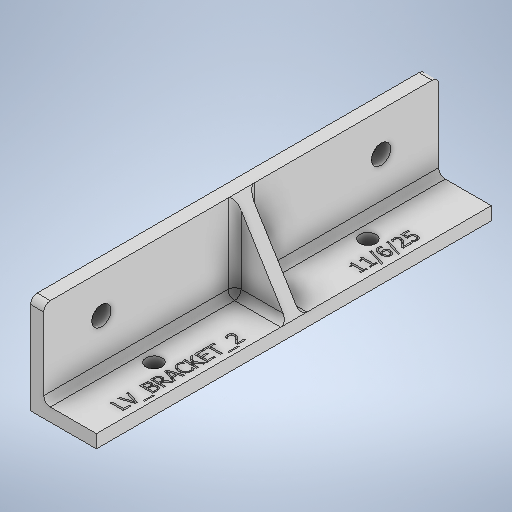
# Autodesk Inventor part: LV_Bracket_2
Saved by Autodesk Inventor 2025 (Build 290162000, 162)
## iProperties
Created: 2025-05-19
Part Number: LV_Bracket_2
Material: Generic
Document SubType Name: Modeling
Designer: mumin
Density: 1 g/cm^3
Appearance: Default
Author: mumin
Autodesk Inventor part; units mm, degrees
ref_plane "YZ Plane" through (0, 0, 0) normal (1, 0, 0) x (0, 1, 0)
ref_plane "XZ Plane" through (0, 0, 0) normal (0, 1, 0) x (-1, 0, 0)
ref_plane "XY Plane" through (0, 0, 0) normal (0, 0, 1) x (1, 0, 0)
sketch "Sketch1" plane through (0, 0, 0) normal (0, 0, 1) x (1, 0, 0)
  line L0 (-4, 26) -> (-4, -4)
  line L1 (-4, -4) -> (16, -4)
  line L2 (16, -4) -> (16, 0)
  line L3 (16, 0) -> (0, 0)
  line L4 (0, 0) -> (0, 26)
  line L5 (0, 26) -> (-4, 26)
  point P0 (0, 0)
  dimension "d0" = 30
  dimension "d1" = 20
  dimension "d2" = 4
  dimension "d3" = 4
  constraints: 12 end point, 5 perpendicular, 1 vertical
  measures "d0" distance of L0.start L0.end
  measures "d1" distance of L0.end L1.end
  measures "d2" distance of L1.end L2.end
  measures "d3" distance between parallel lines of L4 L0
extrude "Base" add sketch "Sketch1" along normal mid plane 120
sketch "Sketch2" plane through (0, 0, 0) normal (0, 0, 1) x (1, 0, 0)
  line L0 (0, 0) -> (0, 26) projected
  line L1 (16, -4) -> (16, 0) projected
  line L2 (0, 26) -> (16, 0)
  line L3 (16, 0) -> (0, 0)
  constraints: 4 end point, 1 perpendicular
extrude "Center Truss" add sketch "Sketch2" along normal mid plane 4
fillet "Fillet1" radius 2 8 edges at (0, 0, 31) (0, 0, -31) (0, 13, 2) (8, 0, 2) (0, 13, -2) (8, 0, -2) (-2, 26, 60) (-2, 26, -60)
sketch "Sketch3" plane through (0, 2, 4) normal (1, 0, 0) x (0, 0, -1)
  line L0 (64, -6) -> (-56, -6) projected
  line L1 (8, 24) -> (0, 24) projected
  point P0 (4, -2)
  point P1 (-38.5, 12.28)
  point P2 (4, 24)
  dimension "d19" = 18.28
  dimension "d20" = 42.5
  constraints: 1 midpoint
  measures "d19" distance from line of L0 point (-38.5, 12.28)
  measures "d20" horizontal distance of point (4, 24) point (-38.5, 12.28)
hole "LV Mount Hole" at (0, 14.28, 42.5) direction (-1, 0, 0) diameter 5.9 depth 4 tip angle 118
mirror "Mirror1" about plane through (0, 0, 0) normal (0, 0, 1) of "LV Mount Hole"
sketch "Sketch4" plane through (2, 0, 4) normal (0, 1, 0) x (1, 0, 0)
  line L0 (14, 0) -> (14, -56) projected
  line L1 (14, 8) -> (14, 0) projected
  point P0 (-2, 4)
  point P1 (4, -28.5)
  point P2 (14, -50)
  point P3 (14, 4)
  dimension "d28" = 10
  dimension "d29" = 32.5
  constraints: 1 midpoint
  measures "d28" distance from line of L0 point (4, -28.5)
  measures "d29" vertical distance of point (14, 4) point (4, -28.5)
hole "80/20 Mount Hole" at (6, 0, 32.5) direction (0, -1, 0) diameter 4.9 depth 4 tip angle 118
mirror "Mirror2" about plane through (0, 0, 0) normal (0, 0, 1) of "80/20 Mount Hole"
sketch "Sketch5" plane through (-4, -4, -60) normal (-1, 0, 0) x (0, 0, 1)
  circle A0 centre (89, 18.28) radius 1.85
  line L0 (120, 28) -> (120, 0) projected
  circle A1 centre (29.5, 18.28) radius 1.85
  circle A2 centre (17.5, 18.28) radius 2.95 projected
  point P0 (60, 4)
  dimension "d31" = 3.7
  dimension "d32" = 31
  dimension "d33" = 3.7
  dimension "d34" = 12
  constraints: 2 centre point
  measures "d31" diameter of A0
  measures "d32" distance from line of L0 A0.centre
  measures "d33" diameter of A1
  measures "d34" distance of A1.centre A2.centre
extrude "Alignment Pins" add sketch "Sketch5" along normal blind 3 contours A0 | A1
fillet "Fillet2" radius 1 2 edges at (-7, 14.28, -32.35) (-7, 14.28, 27.15)
sketch "Sketch6" plane through (2, 0, 60) normal (0, 1, 0) x (1, 0, 0)
  line L0 (7.8938, 9.7827) -> (7.8938, 38.5979) construction
  line L1 (7.8938, 38.5979) -> (11.6186, 38.5979) construction
  line L2 (11.6186, 38.5979) -> (11.6186, 9.7827) construction
  line L3 (11.6186, 9.7827) -> (7.8938, 9.7827) construction
  line L4 (7.6408, 81.9717) -> (7.6408, 104.1889) construction
  line L5 (7.6408, 104.1889) -> (12.6878, 104.1889) construction
  line L6 (12.6878, 104.1889) -> (12.6878, 81.9717) construction
  line L7 (12.6878, 81.9717) -> (7.6408, 81.9717) construction
  line L8 (11.9781, 12.5056) -> (11.9781, 10.1879)
  line L9 (11.9781, 10.1879) -> (7.9781, 10.1879)
  line L10 (7.9781, 10.1879) -> (7.9781, 10.7195)
  line L11 (7.9781, 10.7195) -> (11.5049, 10.7195)
  line L12 (11.5049, 10.7195) -> (11.5049, 12.5056)
  line L13 (11.5049, 12.5056) -> (11.9781, 12.5056)
  line L14 (7.9781, 15.8248) -> (11.9781, 14.4472)
  line L15 (11.9781, 14.4472) -> (11.9781, 13.8735)
  line L16 (11.9781, 13.8735) -> (7.9781, 12.4958)
  line L17 (7.9781, 12.4958) -> (7.9781, 13.0663)
  line L18 (7.9781, 13.0663) -> (11.3006, 14.1749)
  line L19 (11.3006, 14.1749) -> (7.9781, 15.2835)
  line L20 (7.9781, 15.2835) -> (7.9781, 15.8248)
  line L21 (12.782, 18.8459) -> (12.782, 15.76)
  line L22 (12.782, 15.76) -> (12.4352, 15.76)
  line L23 (12.4352, 15.76) -> (12.4352, 18.8459)
  line L24 (12.4352, 18.8459) -> (12.782, 18.8459)
  spline S0 degree 2 poles (10.7496, 21.9221) (11.0478, 21.9221) (11.5049, 21.6952) (11.654, 21.5072) knots 0 0 0 1 2 2 2
  spline S1 degree 2 poles (11.654, 21.5072) (11.829, 21.2803) (11.9781, 20.7649) (11.9781, 20.3564) knots 0 0 0 1 2 2 2
  line L25 (11.9781, 20.3564) -> (11.9781, 19.209)
  line L26 (11.9781, 19.209) -> (7.9781, 19.209)
  line L27 (7.9781, 19.209) -> (7.9781, 20.2689)
  spline S2 degree 2 poles (7.9781, 20.2689) (7.9781, 20.6968) (8.0332, 21.1247) (8.1402, 21.3192) knots 0 0 0 1 2 2 2
  spline S3 degree 2 poles (8.1402, 21.3192) (8.2536, 21.5363) (8.6264, 21.7341) (8.8793, 21.7341) knots 0 0 0 1 2 2 2
  spline S4 degree 2 poles (8.8793, 21.7341) (9.1613, 21.7341) (9.6086, 21.4359) (9.735, 21.1733) knots 0 0 0 1 2 2 2
  line L28 (9.735, 21.1733) -> (9.7545, 21.1733)
  spline S5 degree 2 poles (9.7545, 21.1733) (9.8517, 21.5299) (10.3671, 21.9221) (10.7496, 21.9221) knots 0 0 0 1 2 2 2
  spline S6 degree 2 poles (10.7723, 21.3678) (10.5454, 21.3678) (10.2536, 21.2381) (10.1499, 21.0436) knots 0 0 0 1 2 2 2
  spline S7 degree 2 poles (10.1499, 21.0436) (10.0851, 20.9172) (10.0462, 20.619) (10.0462, 20.3435) knots 0 0 0 1 2 2 2
  line L29 (10.0462, 20.3435) -> (10.0462, 19.7406)
  line L30 (10.0462, 19.7406) -> (11.5243, 19.7406)
  line L31 (11.5243, 19.7406) -> (11.5243, 20.1717)
  spline S8 degree 2 poles (11.5243, 20.1717) (11.5243, 20.5218) (11.4595, 20.9237) (11.3558, 21.0793) knots 0 0 0 1 2 2 2
  spline S9 degree 2 poles (11.3558, 21.0793) (11.2488, 21.2284) (10.983, 21.3678) (10.7723, 21.3678) knots 0 0 0 1 2 2 2
  spline S10 degree 2 poles (8.9538, 21.1798) (8.8112, 21.1798) (8.5972, 21.0825) (8.5357, 20.9756) knots 0 0 0 1 2 2 2
  spline S11 degree 2 poles (8.5357, 20.9756) (8.4643, 20.8459) (8.4319, 20.5315) (8.4319, 20.2495) knots 0 0 0 1 2 2 2
  line L32 (8.4319, 20.2495) -> (8.4319, 19.7406)
  line L33 (8.4319, 19.7406) -> (9.6021, 19.7406)
  line L34 (9.6021, 19.7406) -> (9.6021, 20.3435)
  spline S12 degree 2 poles (9.6021, 20.3435) (9.6021, 20.5931) (9.5502, 20.8297) (9.4692, 20.9561) knots 0 0 0 1 2 2 2
  spline S13 degree 2 poles (9.4692, 20.9561) (9.3914, 21.0793) (9.1418, 21.1798) (8.9538, 21.1798) knots 0 0 0 1 2 2 2
  line L35 (11.9781, 25.5461) -> (11.9781, 24.8556)
  line L36 (11.9781, 24.8556) -> (10.3865, 23.5914)
  line L37 (10.3865, 23.5914) -> (10.3865, 22.982)
  line L38 (10.3865, 22.982) -> (11.9781, 22.982)
  line L39 (11.9781, 22.982) -> (11.9781, 22.4504)
  line L40 (11.9781, 22.4504) -> (7.9781, 22.4504)
  line L41 (7.9781, 22.4504) -> (7.9781, 23.4812)
  spline S14 degree 2 poles (7.9781, 23.4812) (7.9781, 23.8248) (8.0527, 24.2884) (8.1888, 24.4991) knots 0 0 0 1 2 2 2
  spline S15 degree 2 poles (8.1888, 24.4991) (8.325, 24.7098) (8.7496, 24.9529) (9.064, 24.9529) knots 0 0 0 1 2 2 2
  spline S16 degree 2 poles (9.064, 24.9529) (9.5016, 24.9529) (10.0948, 24.5056) (10.2374, 24.1231) knots 0 0 0 1 2 2 2
  line L42 (10.2374, 24.1231) -> (11.9781, 25.5461)
  spline S17 degree 2 poles (9.1062, 24.3986) (8.9311, 24.3986) (8.6621, 24.2754) (8.5746, 24.1457) knots 0 0 0 1 2 2 2
  spline S18 degree 2 poles (8.5746, 24.1457) (8.5, 24.0323) (8.4384, 23.7308) (8.4384, 23.5104) knots 0 0 0 1 2 2 2
  line L43 (8.4384, 23.5104) -> (8.4384, 22.982)
  line L44 (8.4384, 22.982) -> (9.9425, 22.982)
  line L45 (9.9425, 22.982) -> (9.9425, 23.4488)
  spline S19 degree 2 poles (9.9425, 23.4488) (9.9425, 23.679) (9.8614, 24.0453) (9.735, 24.1717) knots 0 0 0 1 2 2 2
  spline S20 degree 2 poles (9.735, 24.1717) (9.6248, 24.2884) (9.3136, 24.3986) (9.1062, 24.3986) knots 0 0 0 1 2 2 2
  line L46 (11.9781, 25.4326) -> (7.9781, 26.7811)
  line L47 (7.9781, 26.7811) -> (7.9781, 27.4359)
  line L48 (7.9781, 27.4359) -> (11.9781, 28.7843)
  line L49 (11.9781, 28.7843) -> (11.9781, 28.2235)
  line L50 (11.9781, 28.2235) -> (10.8598, 27.8605)
  line L51 (10.8598, 27.8605) -> (10.8598, 26.3338)
  line L52 (10.8598, 26.3338) -> (11.9781, 25.9707)
  line L53 (11.9781, 25.9707) -> (11.9781, 25.4326)
  line L54 (10.406, 27.7146) -> (8.5227, 27.0955)
  line L55 (8.5227, 27.0955) -> (10.406, 26.4796)
  line L56 (10.406, 26.4796) -> (10.406, 27.7146)
  spline S21 degree 2 poles (12.0494, 30.726) (12.0494, 30.337) (11.7869, 29.679) (11.5243, 29.4391) knots 0 0 0 1 2 2 2
  spline S22 degree 2 poles (11.5243, 29.4391) (11.265, 29.1992) (10.487, 28.9367) (9.9814, 28.9367) knots 0 0 0 1 2 2 2
  spline S23 degree 2 poles (9.9814, 28.9367) (9.4789, 28.9367) (8.7334, 29.1927) (8.4579, 29.4359) knots 0 0 0 1 2 2 2
  spline S24 degree 2 poles (8.4579, 29.4359) (8.1888, 29.6757) (7.9068, 30.3305) (7.9068, 30.7357) knots 0 0 0 1 2 2 2
  spline S25 degree 2 poles (7.9068, 30.7357) (7.9068, 30.9367) (7.9652, 31.29) (8.0105, 31.4391) knots 0 0 0 1 2 2 2
  spline S26 degree 2 poles (8.0105, 31.4391) (8.0527, 31.5688) (8.1726, 31.8378) (8.2439, 31.9707) knots 0 0 0 1 2 2 2
  line L57 (8.2439, 31.9707) -> (8.8857, 31.9707)
  line L58 (8.8857, 31.9707) -> (8.8857, 31.9286)
  spline S27 degree 2 poles (8.8857, 31.9286) (8.8209, 31.8573) (8.6394, 31.6368) (8.5519, 31.478) knots 0 0 0 1 2 2 2
  spline S28 degree 2 poles (8.5519, 31.478) (8.4676, 31.3256) (8.3606, 30.9658) (8.3606, 30.7325) knots 0 0 0 1 2 2 2
  spline S29 degree 2 poles (8.3606, 30.7325) (8.3606, 30.4764) (8.5713, 30.0193) (8.7723, 29.8475) knots 0 0 0 1 2 2 2
  spline S30 degree 2 poles (8.7723, 29.8475) (8.9765, 29.679) (9.5956, 29.491) (9.9814, 29.491) knots 0 0 0 1 2 2 2
  spline S31 degree 2 poles (9.9814, 29.491) (10.393, 29.491) (10.9862, 29.6887) (11.1904, 29.8605) knots 0 0 0 1 2 2 2
  spline S32 degree 2 poles (11.1904, 29.8605) (11.3882, 30.0291) (11.5891, 30.4796) (11.5891, 30.7325) knots 0 0 0 1 2 2 2
  spline S33 degree 2 poles (11.5891, 30.7325) (11.5891, 30.9626) (11.4757, 31.3548) (11.3914, 31.5072) knots 0 0 0 1 2 2 2
  spline S34 degree 2 poles (11.3914, 31.5072) (11.3071, 31.653) (11.1321, 31.8702) (11.0705, 31.9318) knots 0 0 0 1 2 2 2
  line L59 (11.0705, 31.9318) -> (11.0705, 31.9707)
  line L60 (11.0705, 31.9707) -> (11.7058, 31.9707)
  spline S35 degree 2 poles (11.7058, 31.9707) (11.7674, 31.8378) (11.8809, 31.6044) (11.9327, 31.4391) knots 0 0 0 1 2 2 2
  spline S36 degree 2 poles (11.9327, 31.4391) (11.9911, 31.2641) (12.0494, 30.9658) (12.0494, 30.726) knots 0 0 0 1 2 2 2
  line L61 (11.9781, 35.384) -> (11.9781, 34.6936)
  line L62 (11.9781, 34.6936) -> (10.1175, 33.2316)
  line L63 (10.1175, 33.2316) -> (10.3801, 32.9983)
  line L64 (10.3801, 32.9983) -> (11.9781, 32.9983)
  line L65 (11.9781, 32.9983) -> (11.9781, 32.4667)
  line L66 (11.9781, 32.4667) -> (7.9781, 32.4667)
  line L67 (7.9781, 32.4667) -> (7.9781, 32.9983)
  line L68 (7.9781, 32.9983) -> (9.816, 32.9983)
  line L69 (9.816, 32.9983) -> (7.9781, 34.6385)
  line L70 (7.9781, 34.6385) -> (7.9781, 35.2867)
  line L71 (7.9781, 35.2867) -> (9.7642, 33.6303)
  line L72 (9.7642, 33.6303) -> (11.9781, 35.384)
  line L73 (11.9781, 35.7017) -> (7.9781, 35.7017)
  line L74 (7.9781, 35.7017) -> (7.9781, 38.2041)
  line L75 (7.9781, 38.2041) -> (8.4514, 38.2041)
  line L76 (8.4514, 38.2041) -> (8.4514, 36.2333)
  line L77 (8.4514, 36.2333) -> (9.547, 36.2333)
  line L78 (9.547, 36.2333) -> (9.547, 38.0712)
  line L79 (9.547, 38.0712) -> (10.0203, 38.0712)
  line L80 (10.0203, 38.0712) -> (10.0203, 36.2333)
  line L81 (10.0203, 36.2333) -> (11.5049, 36.2333)
  line L82 (11.5049, 36.2333) -> (11.5049, 38.2041)
  line L83 (11.5049, 38.2041) -> (11.9781, 38.2041)
  line L84 (11.9781, 38.2041) -> (11.9781, 35.7017)
  line L85 (11.9781, 39.7211) -> (8.4514, 39.7211)
  line L86 (8.4514, 39.7211) -> (8.4514, 38.3791)
  line L87 (8.4514, 38.3791) -> (7.9781, 38.3791)
  line L88 (7.9781, 38.3791) -> (7.9781, 41.5947)
  line L89 (7.9781, 41.5947) -> (8.4514, 41.5947)
  line L90 (8.4514, 41.5947) -> (8.4514, 40.2527)
  line L91 (8.4514, 40.2527) -> (11.9781, 40.2527)
  line L92 (11.9781, 40.2527) -> (11.9781, 39.7211)
  line L93 (12.782, 44.6385) -> (12.782, 41.5526)
  line L94 (12.782, 41.5526) -> (12.4352, 41.5526)
  line L95 (12.4352, 41.5526) -> (12.4352, 44.6385)
  line L96 (12.4352, 44.6385) -> (12.782, 44.6385)
  line L97 (11.9781, 47.3548) -> (11.9781, 44.888)
  line L98 (11.9781, 44.888) -> (11.4109, 44.888)
  spline S37 degree 2 poles (11.4109, 44.888) (11.1613, 45.1538) (10.6977, 45.6271) (10.4481, 45.854) knots 0 0 0 1 2 2 2
  spline S38 degree 2 poles (10.4481, 45.854) (9.9457, 46.3111) (9.3428, 46.6449) (9.0219, 46.6449) knots 0 0 0 1 2 2 2
  spline S39 degree 2 poles (9.0219, 46.6449) (8.8533, 46.6449) (8.6005, 46.5412) (8.5194, 46.4472) knots 0 0 0 1 2 2 2
  spline S40 degree 2 poles (8.5194, 46.4472) (8.4384, 46.3532) (8.3574, 46.1068) (8.3574, 45.9577) knots 0 0 0 1 2 2 2
  spline S41 degree 2 poles (8.3574, 45.9577) (8.3574, 45.8151) (8.4287, 45.5234) (8.4838, 45.3905) knots 0 0 0 1 2 2 2
  spline S42 degree 2 poles (8.4838, 45.3905) (8.5292, 45.277) (8.6588, 45.0663) (8.7042, 45.0015) knots 0 0 0 1 2 2 2
  line L99 (8.7042, 45.0015) -> (8.7042, 44.9723)
  line L100 (8.7042, 44.9723) -> (8.1337, 44.9723)
  spline S43 degree 2 poles (8.1337, 44.9723) (8.0527, 45.1376) (7.8938, 45.7308) (7.8938, 45.9966) knots 0 0 0 1 2 2 2
  spline S44 degree 2 poles (7.8938, 45.9966) (7.8938, 46.5574) (8.487, 47.1895) (8.9927, 47.1895) knots 0 0 0 1 2 2 2
  spline S45 degree 2 poles (8.9927, 47.1895) (9.2293, 47.1895) (9.6248, 47.0793) (9.7934, 46.9821) knots 0 0 0 1 2 2 2
  spline S46 degree 2 poles (9.7934, 46.9821) (9.9684, 46.8848) (10.312, 46.6028) (10.4773, 46.4472) knots 0 0 0 1 2 2 2
  spline S47 degree 2 poles (10.4773, 46.4472) (10.7528, 46.1944) (11.3428, 45.5752) (11.5146, 45.3905) knots 0 0 0 1 2 2 2
  line L101 (11.5146, 45.3905) -> (11.5146, 47.3548)
  line L102 (11.5146, 47.3548) -> (11.9781, 47.3548)
  line L103 (11.8191, 84.5292) -> (11.8191, 82.5778)
  line L104 (11.8191, 82.5778) -> (11.4106, 82.5778)
  line L105 (11.4106, 82.5778) -> (11.4106, 83.3039)
  line L106 (11.4106, 83.3039) -> (8.7299, 83.3039)
  line L107 (8.7299, 83.3039) -> (8.7299, 82.5778)
  line L108 (8.7299, 82.5778) -> (8.3636, 82.5778)
  spline S48 degree 2 poles (8.3636, 82.5778) (8.3636, 82.9895) (8.1302, 83.3785) (7.8061, 83.4044) knots 0 0 0 1 2 2 2
  line L109 (7.8061, 83.4044) -> (7.8061, 83.8193)
  line L110 (7.8061, 83.8193) -> (11.4106, 83.8193)
  line L111 (11.4106, 83.8193) -> (11.4106, 84.5292)
  line L112 (11.4106, 84.5292) -> (11.8191, 84.5292)
  line L113 (11.8191, 87.5308) -> (11.8191, 85.5795)
  line L114 (11.8191, 85.5795) -> (11.4106, 85.5795)
  line L115 (11.4106, 85.5795) -> (11.4106, 86.3056)
  line L116 (11.4106, 86.3056) -> (8.7299, 86.3056)
  line L117 (8.7299, 86.3056) -> (8.7299, 85.5795)
  line L118 (8.7299, 85.5795) -> (8.3636, 85.5795)
  spline S49 degree 2 poles (8.3636, 85.5795) (8.3636, 85.9911) (8.1302, 86.3801) (7.8061, 86.406) knots 0 0 0 1 2 2 2
  line L119 (7.8061, 86.406) -> (7.8061, 86.821)
  line L120 (7.8061, 86.821) -> (11.4106, 86.821)
  line L121 (11.4106, 86.821) -> (11.4106, 87.5308)
  line L122 (11.4106, 87.5308) -> (11.8191, 87.5308)
  line L123 (7.6408, 89.9295) -> (12.6878, 88.3639)
  line L124 (12.6878, 88.3639) -> (12.6878, 87.9101)
  line L125 (12.6878, 87.9101) -> (7.6408, 89.4693)
  line L126 (7.6408, 89.4693) -> (7.6408, 89.9295)
  spline S50 degree 2 poles (10.5225, 92.8988) (10.8304, 92.8988) (11.3523, 92.6945) (11.5273, 92.5227) knots 0 0 0 1 2 2 2
  spline S51 degree 2 poles (11.5273, 92.5227) (11.7121, 92.3445) (11.9033, 91.8971) (11.9033, 91.6281) knots 0 0 0 1 2 2 2
  spline S52 degree 2 poles (11.9033, 91.6281) (11.9033, 91.359) (11.7218, 90.915) (11.5403, 90.7464) knots 0 0 0 1 2 2 2
  spline S53 degree 2 poles (11.5403, 90.7464) (11.3231, 90.5389) (10.5938, 90.3056) (10.0622, 90.3056) knots 0 0 0 1 2 2 2
  spline S54 degree 2 poles (10.0622, 90.3056) (9.5403, 90.3056) (8.7007, 90.5195) (8.3896, 90.7432) knots 0 0 0 1 2 2 2
  spline S55 degree 2 poles (8.3896, 90.7432) (8.0849, 90.9603) (7.7445, 91.6475) (7.7445, 92.0981) knots 0 0 0 1 2 2 2
  spline S56 degree 2 poles (7.7445, 92.0981) (7.7445, 92.231) (7.7704, 92.4644) (7.7996, 92.5519) knots 0 0 0 1 2 2 2
  line L127 (7.7996, 92.5519) -> (8.315, 92.5519)
  line L128 (8.315, 92.5519) -> (8.315, 92.5292)
  spline S57 degree 2 poles (8.315, 92.5292) (8.2761, 92.4547) (8.208, 92.1824) (8.208, 92.0268) knots 0 0 0 1 2 2 2
  spline S58 degree 2 poles (8.208, 92.0268) (8.208, 91.5276) (8.8823, 90.915) (9.5435, 90.8566) knots 0 0 0 1 2 2 2
  spline S59 degree 2 poles (9.5435, 90.8566) (9.4106, 91.0479) (9.2648, 91.4498) (9.2648, 91.6897) knots 0 0 0 1 2 2 2
  spline S60 degree 2 poles (9.2648, 91.6897) (9.2648, 91.9231) (9.3588, 92.2731) (9.5014, 92.4644) knots 0 0 0 1 2 2 2
  spline S61 degree 2 poles (9.5014, 92.4644) (9.6667, 92.6848) (10.1789, 92.8988) (10.5225, 92.8988) knots 0 0 0 1 2 2 2
  spline S62 degree 2 poles (10.5451, 92.3542) (10.2988, 92.3542) (9.9649, 92.2245) (9.8482, 92.0819) knots 0 0 0 1 2 2 2
  spline S63 degree 2 poles (9.8482, 92.0819) (9.7639, 91.9749) (9.7088, 91.7091) (9.7088, 91.5697) knots 0 0 0 1 2 2 2
  spline S64 degree 2 poles (9.7088, 91.5697) (9.7088, 91.3817) (9.8223, 91.0284) (9.9293, 90.8566) knots 0 0 0 1 2 2 2
  spline S65 degree 2 poles (9.9293, 90.8566) (9.9876, 90.8534) (10.0978, 90.8469) (10.1821, 90.8469) knots 0 0 0 1 2 2 2
  spline S66 degree 2 poles (10.1821, 90.8469) (10.597, 90.8469) (11.1059, 91.009) (11.2388, 91.1321) knots 0 0 0 1 2 2 2
  spline S67 degree 2 poles (11.2388, 91.1321) (11.3652, 91.2456) (11.4657, 91.4919) (11.4657, 91.6313) knots 0 0 0 1 2 2 2
  spline S68 degree 2 poles (11.4657, 91.6313) (11.4657, 91.9555) (11.0054, 92.3542) (10.5451, 92.3542) knots 0 0 0 1 2 2 2
  line L129 (7.6408, 95.0349) -> (12.6878, 93.4693)
  line L130 (12.6878, 93.4693) -> (12.6878, 93.0154)
  line L131 (12.6878, 93.0154) -> (7.6408, 94.5746)
  line L132 (7.6408, 94.5746) -> (7.6408, 95.0349)
  line L133 (11.8191, 97.9425) -> (11.8191, 95.4757)
  line L134 (11.8191, 95.4757) -> (11.2518, 95.4757)
  spline S69 degree 2 poles (11.2518, 95.4757) (11.0022, 95.7415) (10.5387, 96.2148) (10.2891, 96.4417) knots 0 0 0 1 2 2 2
  spline S70 degree 2 poles (10.2891, 96.4417) (9.7866, 96.8988) (9.1837, 97.2326) (8.8628, 97.2326) knots 0 0 0 1 2 2 2
  spline S71 degree 2 poles (8.8628, 97.2326) (8.6943, 97.2326) (8.4414, 97.1289) (8.3604, 97.0349) knots 0 0 0 1 2 2 2
  spline S72 degree 2 poles (8.3604, 97.0349) (8.2793, 96.9409) (8.1983, 96.6945) (8.1983, 96.5454) knots 0 0 0 1 2 2 2
  spline S73 degree 2 poles (8.1983, 96.5454) (8.1983, 96.4028) (8.2696, 96.1111) (8.3247, 95.9782) knots 0 0 0 1 2 2 2
  spline S74 degree 2 poles (8.3247, 95.9782) (8.3701, 95.8647) (8.4998, 95.654) (8.5451, 95.5892) knots 0 0 0 1 2 2 2
  line L135 (8.5451, 95.5892) -> (8.5451, 95.56)
  line L136 (8.5451, 95.56) -> (7.9746, 95.56)
  spline S75 degree 2 poles (7.9746, 95.56) (7.8936, 95.7253) (7.7348, 96.3185) (7.7348, 96.5843) knots 0 0 0 1 2 2 2
  spline S76 degree 2 poles (7.7348, 96.5843) (7.7348, 97.1451) (8.328, 97.7772) (8.8336, 97.7772) knots 0 0 0 1 2 2 2
  spline S77 degree 2 poles (8.8336, 97.7772) (9.0703, 97.7772) (9.4657, 97.667) (9.6343, 97.5697) knots 0 0 0 1 2 2 2
  spline S78 degree 2 poles (9.6343, 97.5697) (9.8093, 97.4725) (10.1529, 97.1905) (10.3182, 97.0349) knots 0 0 0 1 2 2 2
  spline S79 degree 2 poles (10.3182, 97.0349) (10.5938, 96.7821) (11.1837, 96.1629) (11.3555, 95.9782) knots 0 0 0 1 2 2 2
  line L137 (11.3555, 95.9782) -> (11.3555, 97.9425)
  line L138 (11.3555, 97.9425) -> (11.8191, 97.9425)
  spline S80 degree 2 poles (10.5484, 100.902) (10.8369, 100.902) (11.3296, 100.7172) (11.5111, 100.5487) knots 0 0 0 1 2 2 2
  spline S81 degree 2 poles (11.5111, 100.5487) (11.6926, 100.3801) (11.9033, 99.8777) (11.9033, 99.5665) knots 0 0 0 1 2 2 2
  spline S82 degree 2 poles (11.9033, 99.5665) (11.9033, 99.2812) (11.7769, 98.7237) (11.6764, 98.5195) knots 0 0 0 1 2 2 2
  line L139 (11.6764, 98.5195) -> (11.1092, 98.5195)
  line L140 (11.1092, 98.5195) -> (11.1092, 98.5584)
  spline S83 degree 2 poles (11.1092, 98.5584) (11.1545, 98.62) (11.2712, 98.8501) (11.3231, 98.9895) knots 0 0 0 1 2 2 2
  spline S84 degree 2 poles (11.3231, 98.9895) (11.3782, 99.1483) (11.4398, 99.4109) (11.4398, 99.5762) knots 0 0 0 1 2 2 2
  spline S85 degree 2 poles (11.4398, 99.5762) (11.4398, 99.7383) (11.3231, 100.043) (11.1967, 100.1532) knots 0 0 0 1 2 2 2
  spline S86 degree 2 poles (11.1967, 100.1532) (11.0767, 100.2537) (10.7591, 100.3574) (10.5451, 100.3574) knots 0 0 0 1 2 2 2
  spline S87 degree 2 poles (10.5451, 100.3574) (10.3312, 100.3574) (10.0589, 100.2407) (9.9682, 100.1305) knots 0 0 0 1 2 2 2
  spline S88 degree 2 poles (9.9682, 100.1305) (9.8677, 100.0171) (9.7834, 99.68) (9.7834, 99.4757) knots 0 0 0 1 2 2 2
  spline S89 degree 2 poles (9.7834, 99.4757) (9.7834, 99.2553) (9.8515, 98.8177) (9.8806, 98.6848) knots 0 0 0 1 2 2 2
  line L141 (9.8806, 98.6848) -> (7.8191, 98.6848)
  line L142 (7.8191, 98.6848) -> (7.8191, 100.8793)
  line L143 (7.8191, 100.8793) -> (8.2891, 100.8793)
  line L144 (8.2891, 100.8793) -> (8.2891, 99.2002)
  line L145 (8.2891, 99.2002) -> (9.3555, 99.2002)
  spline S90 degree 2 poles (9.3555, 99.2002) (9.3426, 99.2975) (9.3328, 99.4855) (9.3328, 99.5633) knots 0 0 0 1 2 2 2
  spline S91 degree 2 poles (9.3328, 99.5633) (9.3328, 99.8712) (9.4333, 100.2958) (9.5824, 100.4903) knots 0 0 0 1 2 2 2
  spline S92 degree 2 poles (9.5824, 100.4903) (9.7315, 100.6881) (10.1853, 100.902) (10.5484, 100.902) knots 0 0 0 1 2 2 2
  point P0 (-2, 60)
  constraints: 4 other
emboss "LABEL" sketch "Sketch6" operation cut depth 1 direction (0, -1, 0)
body "Solid1"
